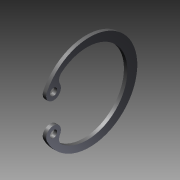
# Autodesk Inventor part: RRING-C-INT-32
Saved by Autodesk Inventor 2011 SP1 (Build 150282100, 282)
## iProperties
Created: 2016-03-21
Part Number: RRING-C-INT-32
Catalog Web Link: www.cadenas.de
Description: RRING_C_INT-Retaining Rings - C  (Internal)
Vendor: MISUMI
Document SubType Name: Modeling
Designer: psAdmin
Manufacturer: MISUMI
Mass: 0.30941 g
Surface Area: 7.54207 cm^2
Volume: 0.30941 cm^3
Density: 1 g/cm^3
Category: PARTsolutions
Company: MISUMI
Title: RRING-C-INT-32
Author: Cadenas PARTsolutions
Comments: Retaining Rings - C  (Internal)
PSOL_IDENT_0: {$CADENAS_DATA\23d-libs\misumi\metric\accessories\rring_c_int.prj},179 {VTYP=3D},{NB=RRING-C-INT-32}
PSOL_IDENT_1: ,{LINA=RRING-C-INT-32},{NN=RRING_C_INT},{DATE=04.08.2015 01:37:13},{GEOMDATE=05.03.2015 00:00:00},{V
PSOL_IDENT_2: ERSION=},{LINEID=170},{LINESUBID=-1},{WBVAR=MAT}  {NB=RRING-C-INT-32},{LINA=RRING-C-INT-32},{KT=DUMM
PSOL_IDENT_3: Y},{PN=RRING-C-INT-32},{TYPE=RRING-C-INT},{MAT=},{HARD=36~44HRC},{NO=32},{DD3=34.4},{DD3TOL=+0.25/-0
PSOL_IDENT_4: .25},{TT=1.20},{TTTOL=+0.06/-0.06},{BB=3.5},{AA=5.2},{DD0=2.5},{DD4=21},{DD1=32},{DD2=33.7},{DD2TOL=
PSOL_IDENT_5: +0.25/0},{MM=1.35},{MMTOL=+0.14/0},{NN=1.5},{A2=12.90}
NN: 1.5
NT: Retaining Rings - C  (Internal)
NB: RRING-C-INT-32
NBSYN: $PN.
LINA: RRING-C-INT-32
PN: RRING-C-INT-32
MAT: Spring Steel
HARD: 36~44HRC
NO: 32
DD3: 34.4
DD3TOL: +0.25/-0.25
TT: 1.20
TTTOL: +0.06/-0.06
BB: 3.5
AA: 5.2
DD0: 2.5
DD4: 21
DD1: 32
DD2: 33.7
DD2TOL: +0.25/0
MM: 1.35
MMTOL: +0.14/0
SUPPLIER: MISUMI
ARTICLENO: RRING-C-INT-32
BOMINFO: RRING-C-INT-32
CREATOR: CADENAS GmbH
Autodesk Inventor part; units mm, degrees
sketch "Sketch_3" plane through (0, 0, 0) normal (1, 0, 0) x (0, 1, 0)
  arc A0 (-15.0884, -7.5008) -> (-15.0884, 7.5008) centre (0, 0) ccw
  arc A1 (-15.0884, 7.5008) -> (-13.5557, 3.9896) centre (-12.8498, 6.3879) ccw
  line L0 (-13.5557, 3.9896) -> (-13.4408, 3.9558)
  arc A2 (-13.4408, 3.9558) -> (-10.45, 7.7412) centre (-12.7067, 6.45) ccw
  arc A3 (-9.83, 11.0525) -> (-10.45, 7.7412) centre (-8.1932, 9.0324) ccw
  arc A4 (-9.83, -11.0525) -> (-9.83, 11.0525) centre (-0.875, 0) ccw
  arc A5 (-10.45, -7.7412) -> (-9.83, -11.0525) centre (-8.1932, -9.0324) ccw
  arc A6 (-10.45, -7.7412) -> (-13.4408, -3.9558) centre (-12.7067, -6.45) ccw
  line L1 (-13.4408, -3.9558) -> (-13.5557, -3.9896)
  arc A7 (-13.5557, -3.9896) -> (-15.0884, -7.5008) centre (-12.8498, -6.3879) ccw
  circle A8 centre (-12.7067, -6.45) radius 1.25
  circle A9 centre (-12.7067, 6.45) radius 1.25
  constraints: 16 point on circle, 10 centre point, 4 end point
extrude "Extrusion1" add sketch "Sketch_3" along normal mid plane 1.2
ref_plane "rr_XY" through (-0.6, 0, 0) normal (1, 0, 0) x (0, 0, -1)
ref_plane "rr_YZ" through (-0.6, 0, 0) normal (0, 0, -1) x (0, 1, 0)
ref_plane "rr_ZX" through (-0.6, 0, 0) normal (0, 1, 0) x (1, 0, 0)
body "Solid1"
